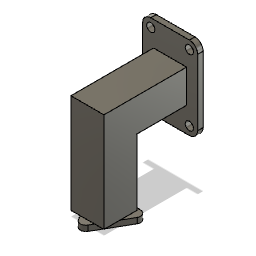
simulation1 (Autodesk Fusion 360 design; units mm, degrees)
Autodesk Fusion 360 part; units mm, degrees
sketch "Sketch1" plane through (0, 0, 0) normal (0, 0, 1) x (1, 0, 0) in component "Mounting Plate1"
  line L0 (-50, 75) -> (50, 75)
  line L1 (50, 75) -> (50, -75)
  line L2 (50, -75) -> (-50, -75)
  line L3 (-50, -75) -> (-50, 75)
  line L4 (-50, 75) -> (50, -75) construction
  line L5 (50, 75) -> (-50, -75) construction
  circle A0 centre (-35, 60) radius 7.5
  circle A1 centre (35, 60) radius 7.5
  line L6 (0, 0) -> (21.7934, 0) construction
  circle A2 centre (-35, -60) radius 7.5
  circle A3 centre (35, -60) radius 7.5
  dimension "d1" = 100
  dimension "d2" = 150
  dimension "d3" = 15
  dimension "d4" = 15
  dimension "d5" = 15
  dimension "d6" = 15
  constraint perpendicular L0 L1
  constraint parallel L0 L2
  constraint parallel L1 L3
  constraint horizontal L0
  constraint coincident L4 L6.start
  constraint coincident L5 L6.start
  constraint coincident L6.start origin
  constraint horizontal L6
  constraint horizontal A0.centre A1.centre
  constraint equal A0 A1
  constraint symmetric A0 L6 A2
  constraint symmetric A1 L6 A3
  measures "d1" distance of L1.end L2.end
  measures "d2" vertical distance of L0.end L1.end
  measures "d3" diameter of A1
  measures "d4" distance of L0 A1.centre
  measures "d5" distance of L1 A1.centre
  measures "d6" distance of L3 A0.centre
extrude "Extrude1" add sketch "Sketch1" along normal blind 10 makes body 1 in component "Mounting Plate1"
fillet "Fillet1" radius 15 4 edges at (-50, 75, 5) (50, 75, 5) (50, -75, 5) (-50, -75, 5) on bodies 1 in component "Mounting Plate1"
ref_plane "WorkPlane1" through (0, -150, 0) normal (0, 1, 0) x (0, 0, 1) in component "Mounting Plate1"
sketch "Sketch2" plane through (0, -150, 0) normal (0, 1, 0) x (1, 0, 0) in component "Mounting Plate1"
  line L0 (-35, -10) -> (35, -10)
  line L1 (0, 0) -> (0, -125) construction
  line L2 (-50, -96.1325) -> (0, -182.735)
  line L3 (0, -182.735) -> (50, -96.1325)
  line L4 (50, -96.1325) -> (-50, -96.1325)
  point P0 (0, -125)
  dimension "d11" = 125
  dimension "d12" = 100
  constraint coincident L1.start origin
  constraint perpendicular L0 L1
  constraint coincident P0 L1.end
  constraint horizontal L4
  measures "d11" vertical distance of L1.start P0
  measures "d12" horizontal distance of L2.start L3.end
extrude "Extrude2" add sketch "Sketch2" against normal blind 10 separate body makes body 2 in component "Mounting Plate1"
fillet "Fillet2" radius 10 3 edges at (0, -155, 182.735) (50, -155, 96.1325) (-50, -155, 96.1325) on bodies 2 in component "Mounting Plate1"
sketch "Sketch1 (2)" plane through (0, 0, 10) normal (0, 0, 1) x (1, 0, 0)
  arc A0 (-50, -60) -> (-35, -75) centre (-35, -60) ccw
  line L0 (-35, -75) -> (35, -75)
  arc A1 (35, -75) -> (50, -60) centre (35, -60) ccw
  line L1 (50, -60) -> (50, 60)
  arc A2 (50, 60) -> (35, 75) centre (35, 60) ccw
  line L2 (35, 75) -> (-35, 75)
  arc A3 (-35, 75) -> (-50, 60) centre (-35, 60) ccw
  line L3 (-50, 60) -> (-50, -60)
  circle A4 centre (35, -60) radius 7.5
  circle A5 centre (-35, 60) radius 7.5
  circle A6 centre (-35, -60) radius 7.5
  circle A7 centre (35, 60) radius 7.5
  line L4 (-30, 30) -> (30, 30)
  line L5 (30, 30) -> (30, -30)
  line L6 (30, -30) -> (-30, -30)
  line L7 (-30, -30) -> (-30, 30)
  line L8 (-30, 30) -> (30, -30) construction
  line L9 (30, 30) -> (-30, -30) construction
  constraint horizontal L4
  constraint perpendicular L4 L5
  constraint parallel L4 L6
  constraint parallel L5 L7
  constraint coincident L8 origin
  constraint coincident L9 origin
extrude "Extrude3" add sketch "Sketch1 (2)" along normal blind 150 contours L4 L5 L6 L7 bodies 1 in component "Mounting Plate1"
sketch "Sketch2 (2)" plane through (0, -30, 0) normal (0, -1, 0) x (1, 0, 0)
  line L0 (-30, 10) -> (30, 10)
  line L1 (30, 10) -> (30, 160)
  line L2 (30, 160) -> (-30, 160)
  line L3 (-30, 160) -> (-30, 10)
  line L4 (-30, 160) -> (30, 160)
  line L5 (30, 160) -> (30, 100)
  line L6 (30, 100) -> (-30, 100)
  line L7 (-30, 100) -> (-30, 160)
  constraint horizontal L4
  constraint vertical L5
  constraint horizontal L6
  constraint vertical L7
  constraint coincident L1 L5.end
  constraint coincident L2.end L3.start
extrude "Extrude4" add sketch "Sketch2 (2)" along normal blind 120 contours L1 L2 L3 L4 L5 L6 L7 bodies 1 2 in component "Mounting Plate1"
component "Mounting Plate1" placed x (1, 0, 0) y (0, 1, 0) z (0, 0, 1) at (0, 0, 0)
equation "d2 = ( 6 * 25 ) * 1 mm"
